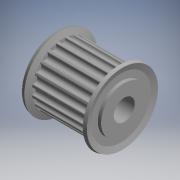
# Autodesk Inventor part: GPA20MR3150-A-HUC_b
Saved by Autodesk Inventor 2017.3 (Build 213256000, 256)
## iProperties
Part Number: GPA20MR3150-A-HUC_b
Material: Generic
Catalog Web Link: www.cadenas.de
Description: GPA__MR3060, GPA__MR3090, GPA__MR3150, GPB__MR3060, GPB__MR3090, GPB__MR3150, GPK__MR3060, GPK__MR3090, GPK__MR3150, GPT__MR3060, GPT__MR3090, GPT__MR3150, GPM__MR3060, GPM__MR3090, GPM__MR3150, GPP__MR3060, GPP__MR3090, GPP__MR3150_body-High Torque Timing Pulleys MR3 Type
Vendor: MISUMI
Document SubType Name: Modeling
Designer: partserver
Manufacturer: MISUMI
Mass: 4.23562 g
Surface Area: 29.4786 cm^2
Volume: 4.23562 cm^3
Density: 1 g/cm^3
Appearance: PSOLRGB-192-192-192
Category: PARTsolutions
Company: MISUMI
Title: GPA20MR3150-A-HUC
Author: Cadenas PARTsolutions
Comments: High Torque Timing Pulleys MR3 Type
PSOL_IDENT_0: {$CADENAS_DATA\23d-libs\misumi\metric\51_timing_pulleys\gpa_mr3\gpa_mr3.prj},583 {VTYP=3D},{NB=GPA20
PSOL_IDENT_1: MR3150-A-HUC_b},{LINA=GPA20MR3150-A-HUC},{NN=GPA__MR3060, GPA__MR3090, GPA__MR3150, GPB__MR3060, GPB
PSOL_IDENT_2: __MR3090, GPB__MR3150, GPK__MR3060, GPK__MR3090, GPK__MR3150, GPT__MR3060, GPT__MR3090, GPT__MR3150,
PSOL_IDENT_3: GPM__MR3060, GPM__MR3090, GPM__MR3150, GPP__MR3060, GPP__MR3090, GPP__MR3150_body},{DATE=08.06.2021
PSOL_IDENT_4: 06:33:48},{GEOMDATE=20.12.2018 05:04:53},{VERSION=},{LINEID=270},{WBVAR=MAT,ST,TNW,PS,SBS,DDM,DDI,Z
PSOL_IDENT_5: ,J,Q,R,S,T,ALT1,ALT2,M,QSC,QFC,QTC,ALT3,K,KSC,KFC,KTC,ALT4,BC,ALT5,ALT6,ALT7,FC,ALT8,TPC,ALT9,SLH},{
PSOL_IDENT_6: WBNUMERIC=DDM,Z,J,Q,R,S,T,QSC,QFC,QTC,K,KSC,KFC,KTC,BC,FC,SLH}  {NB=GPA20MR3150-A-HUC_b},{LINA=GPA20
PSOL_IDENT_7: MR3150-A-HUC},{KT=DUMMY},{PN=GPA20MR3150-A-HUC},{TYPE=GPA},{MAT=AA},{MATALG= 'AA','Aluminum Alloy','
PSOL_IDENT_8: S45C','1045 Carbon Steel' },{ST=CA},{STALG= 'CA','Clear Anodize','BA','Black Anodize','HCA','Hard Cl
PSOL_IDENT_9: ear Anodize' },{NT=20},{TNW=MR3150},{TNWALG= 'MR3060','MR3090','MR3150' },{BW=15},{PS=A},{PSALG= 'A'
PSOL_IDENT_10: ,'K' },{SBS=HU},{SBSALG= 'H','Round Hole','P','Round Hole + Tap','V','Stepped Hole','Y','Both Ends S
PSOL_IDENT_11: tepped Hole','HU','Inch Round Hole' },{DDM=0.00},{DDI=C},{DDMALG=[0]},{DDIALG= 'B','C','D','E' },{DD
PSOL_IDENT_12: HA=[4:4/1],[4.50],[5:6/1],[6.35],[7:10/1]},{DDHBK=[4:4/1],[4.50],[5:6/1],[6.35],[7:8/1]},{DDPA=[4:4/
PSOL_IDENT_13: 1],[4.50],[5:6/1]},{DDPBK=[4:4/1],[4.50],[5:6/1],[6.35],[7:8/1]},{DDNA=},{DDNB=},{DDNK=[10:10/1]},{D
PSOL_IDENT_14: DCA=},{DDCB=},{DDVA=[4:4/1],[4.50],[5:6/1],[6.35],[7:8/1]},{DDVFB=},{DDYA=[4:8/1]},{DDHUA= 'B','C','
PSOL_IDENT_15: D','E' },{DDHUBK= 'B','C','D' },{DDPUA=},{DDPUBK= 'B' },{DDNUA=},{DDNUB=},{IHSN=1/4},{IHSD=6.350},{D
PSOL_IDENT_16: D3D=6.350},{Z=0.0},{ZALG=[0]},{ZMIN=9.000},{ZAMAX=10.000},{ZBMAX=0.000},{DDZ=6.350},{J=0.0},{JALG=0}
PSOL_IDENT_17: ,{JMAX=18.700},{Q=0},{QALG=[0]},{R=0},{RALG=[0]},{QRMIN=9.000},{QRMAX=10.000},{S=0.0},{SALG=[0]},{SM
PSOL_IDENT_18: AX=9.000},{T=0.0},{TALG=[0]},{TMAX=9.000},{SBSPN=-HUC},{A=16.7},{W=20.7},{L=29.0},{PD=19.10},{OD=18.
PSOL_IDENT_19: 34},{D=0},{F=22},{E=14},{DE=14.000},{TT=1},{BBM=0.000},{BBI=0},{BBI3D=0.000},{TT1M=0.000},{TT1I=0.00
PSOL_IDENT_20: 0},{TT1I3D=0.000},{KF=0.000},{KDD=0.000},{TEU=1.140},{TER1=0.910},{TER2=0.280},{ALT1=},{ALT1ALG= '','
PSOL_IDENT_21: Not applicable' },{ANG=126.000},{ALT1PN=},{ALT2=},{ALT2ALG= '','Not applicable' },{M=N/A},{MALG= 'N/
PSOL_IDENT_22: A' },{MFTALG= 'N/A' },{MSALG= 'N/A' },{M3D=0.000},{TAPL=0.000},{KDML=3.900},{ML=3.900},{MUL=0.000},{
PSOL_IDENT_23: PITCH=0.000},{QSC=0.0},{QSCALG=0},{QFC=0.0},{QFCALG=0},{QTC=0.0},{QTCALG=0},{QPCDMIN=0.000},{QPCDMIN
PSOL_IDENT_24: ALG=0.000},{QPCDMAX=10.000},{ALT2PN=},{ALT3=},{ALT3ALG= '','Not applicable' },{K=0.0},{KALG=0},{KMIN=
PSOL_IDENT_25: 4.000},{KFTMAX=0.000},{KSMAX=0.000},{KSC=0.0},{KSCALG=0},{KFC=0.0},{KFCALG=0},{KTC=0.0},{KTCALG=0},{
PSOL_IDENT_26: KPCDMIN=0.000},{KPCDMINALG=0.000},{KPCDMAX=10.000},{ALT3PN=},{ALT4=},{ALT4ALG= '','Not applicable' }
PSOL_IDENT_27: ,{BC=0.0},{BCALG=0},{BCMIN=0.000},{BCMAX=7.800},{WLBC=20.700},{M1WBC=10.350},{ALT4PN=},{ALT5=},{ALT5
PSOL_IDENT_28: ALG= '','w/o Flange not Attached','NFC','with NFC (Flange not Attached)' },{ALT5PN=},{ALT6=},{ALT6AL
PSOL_IDENT_29: G= '','w/o Flange Attached on One Side Only','RFC','with RFC (Flange Attached on The Boss Side Only)'
PSOL_IDENT_30: ,'LFC','with LFC (Flange Attached on The Opposite Side Only)' },{ALT6PN=},{ALT7=},{ALT7ALG= '','w/o
PSOL_IDENT_31: FC (Flange Cut)','FC','with FC (Flange Cut)' },{FC=0.0},{FCALG=0},{FCMIN=19.500},{FCMAX=20.000},{ALT
PSOL_IDENT_32: 7PN=},{ALT8=},{ALT8ALG= '','Not applicable' },{TPC=N/A},{TPCALG= 'N/A' },{TPCM=4.000},{ALT8PN=},{ALT
PSOL_IDENT_33: 9=},{ALT9ALG= '','Not applicable' },{SLH=0},{SLHALG=[0]},{ALT9PN=},{AC=-},{M1=0.000},{M1I=},{M1I3D=0
PSOL_IDENT_34: .0000},{TP=0.000},{M1L=0.000},{M1IL=0.000},{KTT=5.995}
NB: GPA20MR3150-A-HUC_b
NN: GPA__MR3060, GPA__MR3090, GPA__MR3150, GPB__MR3060, GPB__MR3090, GPB__MR3150, GPK__MR3060, GPK__MR3090, GPK__MR3150, GPT__MR3060, GPT__MR3090, GPT__MR3150, GPM__MR3060, GPM__MR3090, GPM__MR3150, GPP__MR3060, GPP__MR3090, GPP__MR3150_body
NT: 20
NBSYN: $PN._b
LINA: GPA20MR3150-A-HUC
CATALOG: Misumi
PN: GPA20MR3150-A-HUC
MAT: Aluminum Alloy
ST: Clear Anodize
TNW: MR3150
BW: 15
PS: A
SBS: Inch Round Hole
DDM: 0
DDI: C
IHSN: 1/4
IHSD: 6.35
Z: 0
J: 0
Q: 0
R: 0
S: 0
T: 0
A: 16.7
W: 20.7
L: 29
PD: 19.1
OD: 18.34
D: 0
F: 22
E: 14
TT: 1
ALT1: Not applicable
ALT2: Not applicable
M: N/A
QSC: 0
QFC: 0
QTC: 0
ALT3: Not applicable
K: 0
KSC: 0
KFC: 0
KTC: 0
ALT4: Not applicable
BC: 0
ALT5: w/o Flange not Attached
ALT6: w/o Flange Attached on One Side Only
ALT7: w/o FC (Flange Cut)
FC: 0
ALT8: Not applicable
TPC: N/A
ALT9: Not applicable
SLH: 0
AC: -
SUPPLIER: MISUMI
ARTICLENO: GPA20MR3150-A-HUC_b
BOMINFO: GPA20MR3150-A-HUC
CREATOR: CADENAS GmbH
Autodesk Inventor part; units mm, degrees
note: some values were not read from the file. Chosen so that the rebuilt part matches the saved one: pattern direction of "Circular Pattern1".
ref_plane "YZ Plane" through (0, 0, 0) normal (1, 0, 0) x (0, 1, 0)
ref_plane "XZ Plane" through (0, 0, 0) normal (0, 1, 0) x (-1, 0, 0)
ref_plane "XY Plane" through (0, 0, 0) normal (0, 0, 1) x (1, 0, 0)
sketch "_____4" plane through (0, 0, 0) normal (0, 0, 1) x (1, 0, 0)
  line L0 (20.7, 0) -> (0, 0)
  line L1 (0, 0) -> (0, 7)
  line L2 (0, 7) -> (1, 7)
  line L3 (1, 7) -> (1, 9.0383)
  line L4 (1, 9.0383) -> (0.5437, 10.7412)
  line L5 (0.5437, 10.7412) -> (1.5097, 11)
  line L6 (1.5097, 11) -> (2, 9.17)
  line L7 (2, 9.17) -> (18.7, 9.17)
  line L8 (18.7, 9.17) -> (19.1903, 11)
  line L9 (19.1903, 11) -> (20.1563, 10.7412)
  line L10 (20.1563, 10.7412) -> (19.7, 9.0383)
  line L11 (19.7, 9.0383) -> (19.7, 7)
  line L12 (19.7, 7) -> (20.7, 7)
  line L13 (20.7, 7) -> (20.7, 0)
  line L14 (20.7, 0) -> (0, 0)
  constraints: 30 end point
revolve "Revolution1" add sketch "_____4" angle 360 about axis through (20.7, 0, 0) along (1, 0, 0)
sketch "_____6" plane through (10.35, 0, 0) normal (1, 0, 0) x (0, 0, -1)
  line L0 (-1.2708, 9.4651) -> (-1.2202, 9.0884)
  arc A0 (-0.9046, 8.8413) -> (-1.2202, 9.0884) centre (-1.183, 8.8109) ccw
  arc A1 (-0.9046, 8.8413) -> (0.9046, 8.8413) centre (0, 8.94) ccw
  arc A2 (1.2202, 9.0884) -> (0.9046, 8.8413) centre (1.183, 8.8109) ccw
  line L1 (1.2202, 9.0884) -> (1.2708, 9.4651)
  arc A3 (1.2708, 9.4651) -> (-1.2708, 9.4651) centre (0, 0) ccw
  constraints: 8 point on circle, 4 centre point, 4 end point
extrude "Extrusion1" cut sketch "_____6" along normal mid plane 16.7
pattern_circular "Circular Pattern1" count 20 over 360 about axis through (10.35, 0, 0) along (1, 0, 0) of "Extrusion1"
sketch "Sketch3" plane through (20.7, 0, 0) normal (1, 0, 0) x (0, 0, -1)
  point P0 (0, 0)
hole "Hole1" at (20.7, 0, 0) direction (-1, 0, 0) diameter 6.35 depth 20.7
body "Solid1"
